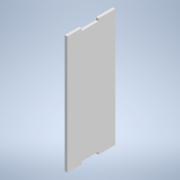
# Autodesk Inventor part: dak
Saved by Autodesk Inventor 2021 (Build 250183000, 183)
## iProperties
Created: 2022-02-02
Part Number: dak
Material: Generic
Document SubType Name: Modeling
Designer: ryan
Density: 1 g/cm^3
Appearance: Default
Author: ryan
Autodesk Inventor part; units mm, degrees
ref_plane "YZ Plane" through (0, 0, 0) normal (1, 0, 0) x (0, 1, 0)
ref_plane "XZ Plane" through (0, 0, 0) normal (0, 1, 0) x (-1, 0, 0)
ref_plane "XY Plane" through (0, 0, 0) normal (0, 0, 1) x (1, 0, 0)
sketch "Sketch1" plane through (0, 0, 0) normal (1, 0, 0) x (0, 1, 0)
  line L0 (0, 0) -> (0, 20)
  line L1 (0, 0) -> (-70, 0)
  line L2 (-70, 0) -> (-70, 57)
  line L3 (-70, 57) -> (0, 57)
  line L4 (0, 57) -> (0, 0)
  line L5 (0, 0) -> (-3, 0)
  line L6 (-3, 0) -> (-3, 20)
  line L7 (-3, 20) -> (0, 20)
  line L8 (0, 20) -> (0, 0)
  line L9 (-3, 20) -> (0, 20)
  line L10 (0, 20) -> (0, 40)
  line L11 (0, 40) -> (-3, 40)
  line L12 (-3, 40) -> (-3, 20)
  line L13 (-3, 40) -> (-3, 57)
  line L14 (0, 40) -> (0, 57)
  dimension "d0" = 20
  dimension "d1" = 70
  dimension "d2" = 57
  dimension "d3" = 3
  dimension "d4" = 20
  dimension "d5" = 3
  dimension "d6" = 20
  constraints: 30 end point, 6 parallel, 4 perpendicular, 3 horizontal, 1 point on line, 1 vertical
  measures "d0" distance of L0.start L0.end
  measures "d1" distance of L2.end L3.end
  measures "d2" distance of L1.end L2.end
  measures "d3" distance of L6.end L7.end
  measures "d4" distance of L5.end L6.end
  measures "d5" distance of L11.end L10.end
  measures "d6" distance of L10.end L9.end
extrude "Extrusion1" add sketch "Sketch1" against normal blind 3 contours L1 L6 L7 L0 | L1 L2 L3 L13 L12 L6 | L11 L13 L3 L4
mirror "Mirror1" about plane through (0, -70, 0) normal (0, -1, 0) of "Extrusion1"
body "Solid1"
